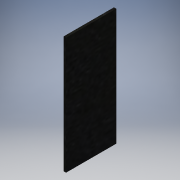
# Autodesk Inventor part: upper insert
Saved by Autodesk Inventor 2019 (Build 230136000, 136)
## iProperties
Created: 2020-03-06
Part Number: upper insert
Material: Generic
Document SubType Name: Modeling
Designer: ntb11189
Density: 1 g/cm^3
Appearance: Smooth - Black
Author: ntb11189
Autodesk Inventor part; units mm, degrees
ref_plane "YZ Plane" through (0, 0, 0) normal (1, 0, 0) x (0, 1, 0)
ref_plane "XZ Plane" through (0, 0, 0) normal (0, 1, 0) x (-1, 0, 0)
ref_plane "XY Plane" through (0, 0, 0) normal (0, 0, 1) x (1, 0, 0)
sketch "Sketch1" plane through (0, 0, 0) normal (1, 0, 0) x (0, 1, 0)
  line L0 (0, 0) -> (-116.5, 0)
  line L1 (-116.5, 0) -> (-116.5, -50)
  line L2 (-116.5, -50) -> (0, -50)
  line L3 (0, -50) -> (0, 0)
  dimension "d0" = 116.5
  dimension "d1" = 50
  constraints: 8 end point, 2 parallel, 1 horizontal, 1 perpendicular
  measures "d0" distance of L2.end L1.end
  measures "d1" distance of L0.end L1.end
extrude "Extrusion1" add sketch "Sketch1" along normal blind 2.3
body "Solid1"
